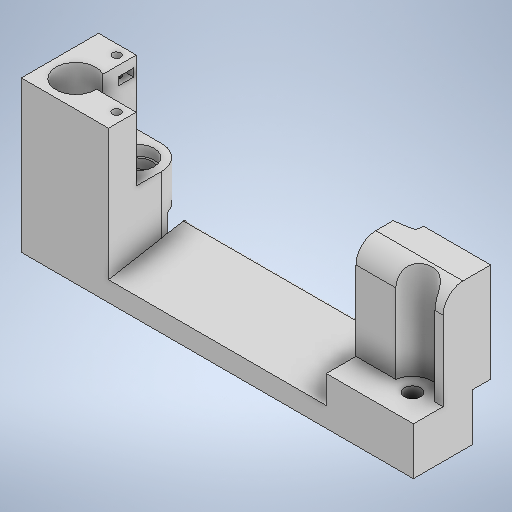
# Autodesk Inventor part: 13042026-16
Saved by Autodesk Inventor 2025.2 (Build 292293000, 293)
## iProperties
Created: 2026-05-27
Part Number: 13042026-16
Material: Generic
Document SubType Name: Modeling
Designer: Oski
Density: 1 g/cm^3
Appearance: Default
Author: Oski
Autodesk Inventor part; units mm, degrees
ref_plane "YZ Plane" through (0, 0, 0) normal (1, 0, 0) x (0, 1, 0)
ref_plane "XZ Plane" through (0, 0, 0) normal (0, 1, 0) x (-1, 0, 0)
ref_plane "XY Plane" through (0, 0, 0) normal (0, 0, 1) x (1, 0, 0)
sketch "Sketch1" plane through (0, 0, 0) normal (0, 0, 1) x (1, 0, 0)
  line L0 (-99, 12) -> (99, 12)
  line L1 (99, 12) -> (99, -12)
  line L2 (99, -12) -> (-99, -12)
  line L3 (-99, -12) -> (-99, 12)
  line L4 (-99, 12) -> (99, -12) construction
  line L5 (99, 12) -> (-99, -12) construction
  point P0 (0, 0)
  dimension "d0" = 24
  dimension "d1" = 198
  constraints: 12 end point, 2 midpoint, 2 parallel, 1 horizontal, 1 perpendicular
  measures "d0" distance of L0.end L1.end
  measures "d1" distance of L0.start L0.end
extrude "Extrusion1" add sketch "Sketch1" along normal blind 30
sketch "Sketch2" plane through (-99, 12, 0) normal (0, 1, 0) x (1, 0, 0)
  line L0 (0, 0) -> (0, -30) projected
  line L1 (0, -15) -> (198, -15)
  line L2 (198, -15) -> (198, 9)
  line L3 (198, 9) -> (0, 9)
  line L4 (0, 9) -> (0, -15)
  line L5 (198, 0) -> (198, -30) projected
  line L6 (198, 0) -> (0, 0) projected
  point P0 (99, 0)
  dimension "d4" = 9
  constraints: 8 end point, 2 midpoint, 2 parallel, 1 horizontal, 1 perpendicular
  measures "d4" distance between parallel lines of L3 L6
extrude "Extrusion2" add sketch "Sketch2" along normal blind 50
fillet "Fillet1" radius 10 1 edges at (0, 62, 15)
sketch "Sketch4" plane through (-99, -12, 0) normal (0, -1, 0) x (1, 0, 0)
  line L0 (198, 16.5) -> (0, 16.5) construction
  line L1 (0, 0) -> (0, 30) projected
  line L2 (198, 0) -> (198, 30) projected
  line L3 (0, 30) -> (198, 30) projected
  line L4 (14, 25) -> (184, 25)
  line L5 (14, 8) -> (184, 8)
  arc A0 (184, 8) -> (184, 25) centre (184, 16.5) ccw
  arc A1 (14, 25) -> (14, 8) centre (14, 16.5) ccw
  line L6 (14, 16.5) -> (0, 16.5)
  line L7 (184, 16.5) -> (198, 16.5)
  point P0 (99, 0)
  point P1 (98, 16.5)
  point P2 (126, 16.5)
  point P3 (182, 16.5)
  point P4 (70, 16.5)
  dimension "d23" = 56
  dimension "d24" = 28
  dimension "d27" = 28
  dimension "d28" = 56
  dimension "d37" = 17
  dimension "d38" = 170
  dimension "d47" = 5
  constraints: 10 end point, 9 point on line, 4 point on circle, 3 horizontal, 3 tangent, 2 centre point, 2 equal length, 2 perpendicular
  measures "d23" distance of point (126, 16.5) point (182, 16.5)
  measures "d24" distance of point (98, 16.5) point (126, 16.5)
  measures "d27" distance of point (70, 16.5) point (98, 16.5)
  measures "d28" distance of L6.start point (70, 16.5)
  measures "d37" distance between parallel lines of L5 L4
  measures "d38" distance of L7.start L6.start
  measures "d47" distance between parallel lines of L3 L4
extrude "Extrusion3" cut sketch "Sketch4" against normal blind 8 contours A1 L4 A0 L5
sketch "Sketch6" plane through (-99, 62, 0) normal (0, 1, 0) x (1, 0, 0)
  line L0 (198, 9) -> (0, 9) projected
  line L1 (198, -15) -> (0, -15) projected
  line L2 (44, 9) -> (154, 9)
  line L3 (154, 9) -> (154, -30)
  line L4 (154, -30) -> (44, -30)
  line L5 (44, -30) -> (44, 9)
  line L6 (44, -5) -> (0, -5)
  line L7 (0, 0) -> (0, -30) projected
  line L8 (154, -5) -> (198, -5)
  line L9 (198, -5) -> (198, 9) projected
  line L10 (44, -5) -> (44, -5)
  point P0 (99, 0)
  point P1 (154, 9)
  point P2 (198, -30)
  dimension "d44" = 110
  dimension "d74" = 0
  constraints: 14 end point, 7 point on line, 2 horizontal, 2 parallel, 2 perpendicular, 1 collinear
  measures "d44" distance between parallel lines of L3 L5
  measures "d74" distance of L6.start L10.end
extrude "Extrusion5" cut sketch "Sketch6" against normal blind 64 contours L3 L1 L5 L0 | L3 L4 L5 L1
sketch "Sketch7" plane through (-99, 62, 0) normal (0, 1, 0) x (1, 0, 0)
  line L0 (0, -15) -> (0, -30) projected
  line L1 (44, 9) -> (0, 9)
  line L2 (0, 9) -> (0, -15)
  line L3 (0, -15) -> (44, -15)
  line L4 (44, -15) -> (44, 9)
  point P0 (99, 0)
  constraints: 8 end point, 2 parallel, 1 horizontal, 1 perpendicular
extrude "Extrusion6" cut sketch "Sketch7" against normal blind 30
sketch "Sketch13" plane through (-99, 32, 0) normal (0, 1, 0) x (1, 0, 0)
  line L0 (0, 9) -> (44, 9) projected
  line L1 (0, -15) -> (0, 9) projected
  point P0 (99, 0)
  point P1 (32, -3)
  dimension "d79" = 12
  dimension "d80" = 32
  measures "d79" distance from line of L0 point (32, -3)
  measures "d80" distance from line of L1 point (32, -3)
hole "Hole5" at (-67, 32, 3) direction (0, -1, 0) diameter 14.2 depth 10 counterbore diameter 16.2 counterbore depth 5.2
sketch "Sketch14" plane through (-99, 32, 0) normal (0, 1, 0) x (1, 0, 0)
  line L0 (0, -15) -> (0, -30) projected
  line L1 (44, 9) -> (0, 9) projected
  line L2 (0, -15) -> (19, -15)
  line L3 (19, -15) -> (19, 9)
  line L4 (19, 9) -> (0, 9)
  line L5 (0, 9) -> (0, -15)
  line L6 (44, -15) -> (0, -15) projected
  line L7 (44, -15) -> (35, -15)
  line L8 (44, -1.2) -> (44, -15)
  point P0 (99, 0)
  dimension "d88" = 19
  constraints: 12 end point, 2 horizontal, 2 parallel, 1 perpendicular, 1 point on line
  measures "d88" distance of L0.start L2.end
extrude "Extrusion9" add sketch "Sketch14" along normal blind 32.3
sketch "Sketch16" plane through (-55, -2, 0) normal (1, 0, 0) x (0, 0, -1)
  line L0 (-30, 0) -> (-30, 14) projected
  line L1 (-30, 0) -> (9, 7)
  line L2 (9, 14) -> (0, 14) projected
  line L3 (9, 7) -> (9, 0)
  line L4 (-30, 0) -> (9, 0)
  point P0 (0, 2)
  point P1 (-30, -5)
  point P2 (0, 0)
  dimension "d94" = 7
  dimension "d95" = 9
  constraints: 6 end point, 1 point on line, 1 vertical
  measures "d94" distance from line of L1.end L2
  measures "d95" distance from line of point (0, 0) L3
extrude "Extrusion10" add sketch "Sketch16" along normal blind 110
fillet "Fillet2" radius 1 1 edges at (0, 5, -9)
fillet "Fillet3" radius 12 1 edges at (-55, 22, -9)
sketch "Sketch17" plane through (-99, 62, 0) normal (0, 1, 0) x (1, 0, 0)
  line L0 (154, 9) -> (162, 9)
  line L1 (162.3147, 5.0249) -> (154, 3.7)
  line L2 (154, 3.7) -> (154, 9)
  arc A0 (162.3147, 5.0249) -> (164, 7) centre (162, 7) ccw
  line L3 (164, 2.3546) -> (164, 11.6454) construction
  line L4 (164, 7) -> (164, 9)
  line L5 (164, 9) -> (162, 9)
  point P0 (99, 0)
  dimension "d102" = 2
  dimension "d103" = 10
  dimension "d104" = 5.3
  constraints: 12 end point, 3 tangent, 2 point on circle, 2 vertical, 1 centre point, 1 coincident, 1 collinear, 1 horizontal, 1 midpoint, 1 point on line
  measures "d102" radius of A0
  measures "d103" distance between parallel lines of L3 L2
  measures "d104" distance of L1.end L0.start
extrude "Extrusion11" cut sketch "Sketch17" against normal blind 110
sketch "Sketch18" plane through (-99, 12, 30) normal (0, 1, 0) x (1, 0, 0)
  line L0 (44, 0) -> (44, 27) projected
  line L1 (44, 14) -> (0, 14)
  line L2 (0, 14) -> (0, 0)
  line L3 (0, 0) -> (44, 0)
  line L4 (44, 0) -> (44, 14)
  line L5 (44, 15) -> (0, 15) projected
  line L6 (0, 15) -> (0, 0) projected
  line L7 (44, 0) -> (0, 0) projected
  line L8 (0, 14) -> (19, 14)
  line L9 (19, 14) -> (19, 15)
  line L10 (19, 15) -> (0, 15)
  line L11 (0, 15) -> (0, 14)
  point P0 (99, 30)
  point P1 (44, 14)
  point P2 (0, 15)
  point P3 (0, 14)
  point P4 (0, 14)
  point P5 (0, 14)
  dimension "d109" = 1
  constraints: 16 end point, 5 point on line, 4 parallel, 2 horizontal, 2 perpendicular
  measures "d109" distance between parallel lines of L5 L1
extrude "Extrusion13" add sketch "Sketch18" along normal blind 52.3 contours L3 L2 L1 L0 | L1 L6 L5 L9
sketch "Sketch19" plane through (-80, 12, 15) normal (0, 1, 0) x (1, 0, 0)
  line L0 (25, 0) -> (0, 0) projected
  line L1 (0, -1) -> (25, -1) projected
  line L2 (0, 0) -> (25, 0)
  line L3 (25, 0) -> (25, -1)
  line L4 (25, -1) -> (0, -1)
  line L5 (0, -1) -> (0, 0)
  point P0 (80, 15)
  constraints: 8 end point, 2 parallel, 1 horizontal, 1 perpendicular
extrude "Extrusion14" add sketch "Sketch19" along normal blind 20
sketch "Sketch20" plane through (-99, 64.3, 0) normal (0, 1, 0) x (1, 0, 0)
  line L0 (14.1654, 3.9806) -> (38.9806, -20.8346) construction
  circle A0 centre (32, -3) radius 8.1 construction
  circle A1 centre (32, -3) radius 8.1 construction
  line L1 (26.573, -8.427) -> (32, -3) construction
  line L2 (14.1654, 3.9806) -> (14.1654, 9) construction
  line L3 (32, 9) -> (0, 9) construction
  line L4 (38.9806, -20.8346) -> (44, -20.8346) construction
  line L5 (44, -30) -> (44, -16) construction
  point P0 (99, 0)
  dimension "d114" = 35.094
  dimension "d116" = 7.675
  constraints: 8 end point, 2 concentric, 2 perpendicular, 2 point on line, 1 centre point, 1 coincident, 1 horizontal, 1 midpoint, 1 vertical
  measures "d114" distance of L0.start L0.end
  measures "d116" distance of L1.start L1.end
hole "Hole6" at (-84.8346, 64.3, -3.9806) at (-60.0194, 64.3, 20.8346) direction (0, -1, 0) diameter 4.2 depth 16
sketch "Sketch21" plane through (-99, -12, 0) normal (0, -1, 0) x (1, 0, 0)
  line L0 (0, 0) -> (0, 30) projected
  line L1 (0, 0) -> (198, 0) projected
  line L2 (198, 0) -> (198, 30) projected
  point P0 (99, 0)
  point P1 (14, 16.5)
  point P2 (184, 16.5)
  dimension "d124" = 14
  dimension "d125" = 16.5
  dimension "d126" = 16.5
  dimension "d127" = 14
  measures "d124" distance from line of L0 point (14, 16.5)
  measures "d125" distance from line of L1 point (14, 16.5)
  measures "d126" distance from line of L1 point (184, 16.5)
  measures "d127" distance from line of L2 point (184, 16.5)
hole "Hole7" at (-85, -12, 16.5) at (85, -12, 16.5) direction (0, 1, 0) diameter 8.2 end through all
sketch "Sketch22" plane through (-99, 64.3, 0) normal (0, 1, 0) x (1, 0, 0)
  circle A0 centre (184, -16.5) radius 10
  circle A1 centre (14, -16.5) radius 10
  arc A2 (180.1842, -15) -> (187.8158, -15) centre (184, -16.5) ccw projected
  circle A3 centre (14, -16.5) radius 4.1 projected
  point P0 (99, 0)
  dimension "d135" = 20
  dimension "d136" = 20
  constraints: 2 centre point, 2 concentric
  measures "d135" diameter of A0
  measures "d136" diameter of A1
extrude "Extrusion15" cut sketch "Sketch22" against normal blind 52.3 contours A0 | A1 | A3
sketch "Sketch23" plane through (-99, -4, 0) normal (0, -1, 0) x (1, 0, 0)
  circle A0 centre (14, 16.5) radius 10
  circle A1 centre (14, 16.5) radius 4.1 projected
  circle A2 centre (184, 16.5) radius 10
  circle A3 centre (184, 16.5) radius 4.1 projected
  point P0 (99, 0)
  dimension "d139" = 20
  dimension "d140" = 20
  constraints: 2 centre point, 2 concentric
  measures "d139" diameter of A0
  measures "d140" diameter of A2
extrude "Extrusion16" add sketch "Sketch23" along normal blind 8
sketch "Sketch24" plane through (0, 0, 16) normal (0, 0, 1) x (1, 0, 0)
  line L0 (-62.1194, 64.3) -> (-57.9194, 64.3) projected
  line L1 (-60.0194, 64.3) -> (-60.0194, 57.3) construction
  line L2 (-63.7694, 59.3) -> (-56.2694, 59.3)
  line L3 (-56.2694, 59.3) -> (-56.2694, 55.3)
  line L4 (-56.2694, 55.3) -> (-63.7694, 55.3)
  line L5 (-63.7694, 55.3) -> (-63.7694, 59.3)
  line L6 (-63.7694, 59.3) -> (-56.2694, 55.3) construction
  line L7 (-56.2694, 59.3) -> (-63.7694, 55.3) construction
  point P0 (0, 0)
  dimension "d143" = 7
  dimension "d144" = 7.5
  dimension "d145" = 4
  constraints: 14 end point, 3 midpoint, 2 parallel, 1 horizontal, 1 perpendicular, 1 vertical
  measures "d143" distance of L1.start L1.end
  measures "d144" distance of L2.start L2.end
  measures "d145" distance of L4.end L2.start
sketch "Sketch25" plane through (-80, -12, 0) normal (-1, 0, 0) x (0, 0, 1)
  line L0 (-6.0806, 76.3) -> (-1.8806, 76.3) projected
  line L1 (-3.9806, 76.3) -> (-3.9806, 69.3) construction
  line L2 (-7.7306, 71.3) -> (-0.2306, 71.3)
  line L3 (-0.2306, 71.3) -> (-0.2306, 67.3)
  line L4 (-0.2306, 67.3) -> (-7.7306, 67.3)
  line L5 (-7.7306, 67.3) -> (-7.7306, 71.3)
  line L6 (-7.7306, 71.3) -> (-0.2306, 67.3) construction
  line L7 (-0.2306, 71.3) -> (-7.7306, 67.3) construction
  point P0 (0, 12)
  dimension "d146" = 7
  dimension "d147" = 7.5
  dimension "d148" = 4
  constraints: 14 end point, 3 midpoint, 2 parallel, 1 horizontal, 1 perpendicular, 1 vertical
  measures "d146" distance of L1.start L1.end
  measures "d147" distance of L2.start L2.end
  measures "d148" distance of L4.end L2.start
extrude "Extrusion17" cut sketch "Sketch25" along normal blind 9
extrude "Extrusion18" cut sketch "Sketch24" along normal blind 9
body "Solid1"
